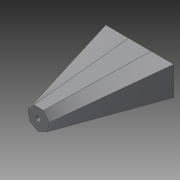
# Autodesk Inventor part: Part2
Saved by Autodesk Inventor 2015 (Build 190159000, 159)
## iProperties
Created: 2015-01-27
Part Number: Part2
Material: Generic
Document SubType Name: Modeling
Designer: PLTW-Stu-02
Density: 1 g/cm^3
Appearance: Default
Author: PLTW-Stu-02
Autodesk Inventor part; units mm, degrees
ref_plane "YZ Plane" through (0, 0, 0) normal (1, 0, 0) x (0, 1, 0)
ref_plane "XZ Plane" through (0, 0, 0) normal (0, 1, 0) x (-1, 0, 0)
sketch "Sketch1" plane through (0, 0, 0) normal (0, 0, 1) x (1, 0, 0)
  line L0 (8.7133, 24.8361) -> (43.4393, 24.8361)
  line L1 (43.4393, 24.8361) -> (43.4393, 10.1443)
  line L2 (43.4393, 10.1443) -> (8.7133, 10.1443)
  line L3 (8.7133, 10.1443) -> (8.7133, 24.8361)
  point P0 (0, 0)
  constraints: 8 end point, 2 parallel, 1 horizontal, 1 perpendicular
ref_plane "Work Plane1" through (0, 0, 50.8) normal (0, 0, 1) x (1, 0, 0)
sketch "Sketch2" plane through (0, 0, 50.8) normal (0, 0, 1) x (1, 0, 0)
  line L0 (29.514, 13.3941) -> (25.0936, 11.3585)
  line L1 (25.0936, 11.3585) -> (20.746, 13.5453)
  line L2 (20.746, 13.5453) -> (19.745, 18.3079)
  line L3 (19.745, 18.3079) -> (22.8445, 22.0599)
  line L4 (22.8445, 22.0599) -> (27.7104, 21.976)
  line L5 (27.7104, 21.976) -> (30.6786, 18.1193)
  line L6 (30.6786, 18.1193) -> (29.514, 13.3941)
  point P0 (0, 0)
  point P1 (25.1903, 16.9659)
  constraints: 14 end point, 15 other
loft "Loft1" add profiles "Sketch1", "Sketch2"
hole "Hole1" at (25.0277, 16.9659, 50.8) direction (0, 0, -1) diameter 1.778 depth 9.525 tip angle 118 countersink diameter 2.54 countersink angle 82
body "Solid1"
